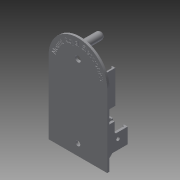
# Autodesk Inventor part: Robot Chassis(V2)7.stl
Saved by Autodesk Inventor 2015 SP1 (Build 190203100, 203)
## iProperties
Created: 2014-11-28
Part Number: Robot Chassis(V2)7.stl
Material: Generic
Document SubType Name: Modeling
Designer: shmyrk
Density: 1 g/cm^3
Appearance: Default
Author: shmyrk
Autodesk Inventor part; units mm, degrees
ref_plane "YZ Plane" through (0, 0, 0) normal (1, 0, 0) x (0, 1, 0)
ref_plane "XZ Plane" through (0, 0, 0) normal (0, 1, 0) x (-1, 0, 0)
ref_plane "XY Plane" through (0, 0, 0) normal (0, 0, 1) x (1, 0, 0)
sketch "Sketch1" plane through (0, 0, 0) normal (0, 1, 0) x (-1, 0, 0)
  line L0 (0, 0) -> (80, 0)
  line L1 (80, 0) -> (80, 100)
  line L2 (0, 100) -> (0, 0)
  arc A0 (80, 100) -> (0, 100) centre (40, 100) ccw
  dimension "d1" = 100
  dimension "d178" = 40
  dimension "d179" = 100
  dimension "d180" = 80
  constraints: 6 end point, 2 point on circle, 1 centre point, 1 horizontal, 1 parallel, 1 perpendicular
  measures "d1" distance of L1.end L0.end
  measures "d178" radius of A0
  measures "d179" distance from line of L0 A0.centre
  measures "d180" distance of L0.start L0.end
extrude "Extrusion1" add sketch "Sketch1" along normal blind 3
sketch "Sketch2" plane through (0, 3, 0) normal (0, 1, 0) x (1, 0, 0)
  line L0 (-80, -20) -> (-77, -20)
  line L1 (-77, -20) -> (-77, -56)
  line L2 (-77, -56) -> (-80, -56)
  line L3 (-80, -56) -> (-80, -20)
  line L4 (-3, -20) -> (0, -20)
  line L5 (0, -20) -> (0, -56)
  line L6 (0, -56) -> (-3, -56)
  line L7 (-3, -56) -> (-3, -20)
  line L8 (-77, -20) -> (-58, -20)
  line L9 (-3, -20) -> (-22, -20)
  line L10 (-58, -20) -> (-55, -20)
  line L11 (-55, -20) -> (-55, -56)
  line L12 (-55, -56) -> (-58, -56)
  line L13 (-58, -56) -> (-58, -20)
  line L14 (-25, -20) -> (-22, -20)
  line L15 (-22, -20) -> (-22, -56)
  line L16 (-22, -56) -> (-25, -56)
  line L17 (-25, -56) -> (-25, -20)
  line L18 (-80, -20) -> (-80, -20)
  line L19 (-80, 0) -> (-80, -100) projected
  line L20 (-80, -20) -> (-80, 0)
  line L21 (-80, 0) -> (-80, -100) projected
  line L22 (0, 0) -> (0, -100)
  arc A0 (-80, -100) -> (0, -100) centre (-40, -100) ccw projected
  line L23 (0, -20) -> (0, -20)
  dimension "d5" = 3
  dimension "d7" = 3
  dimension "d9" = 19
  dimension "d10" = 19
  dimension "d11" = 3
  dimension "d13" = 3
  dimension "d117" = 0
  dimension "d118" = 20
  dimension "d120" = 0
  dimension "d126" = 36
  constraints: 44 end point, 8 parallel, 6 collinear, 6 perpendicular, 5 horizontal, 2 point on line, 1 coincident, 1 tangent, 1 vertical
  measures "d5" distance of L1.end L2.end
  measures "d7" distance of L5.end L6.end
  measures "d9" distance of L8.end L0.end
  measures "d10" distance of L9.end L4.start
  measures "d11" distance of L11.end L12.end
  measures "d13" distance of L16.start L16.end
  measures "d117" distance of L0.start L18.end
  measures "d118" distance of L18.end L19.start
  measures "d120" distance of L23.start L4.end
  measures "d126" distance of L16.end L17.end
extrude "Extrusion2" add sketch "Sketch2" along normal blind 7
sketch "Sketch3" plane through (0, 10, 0) normal (0, 1, 0) x (1, 0, 0)
  line L0 (-80, -20) -> (-77, -20)
  line L1 (-77, -20) -> (-77, -41)
  line L2 (-77, -41) -> (-80, -41)
  line L3 (-80, -41) -> (-80, -20)
  line L4 (-3, -20) -> (0, -20)
  line L5 (0, -20) -> (0, -41)
  line L6 (0, -41) -> (-3, -41)
  line L7 (-3, -41) -> (-3, -20)
  line L8 (-58, -20) -> (-55, -20)
  line L9 (-55, -20) -> (-55, -41)
  line L10 (-55, -41) -> (-58, -41)
  line L11 (-58, -41) -> (-58, -20)
  line L12 (-25, -20) -> (-22, -20)
  line L13 (-22, -20) -> (-22, -41)
  line L14 (-22, -41) -> (-25, -41)
  line L15 (-25, -41) -> (-25, -20)
  point P0 (0, 0)
  dimension "d17" = 21
  dimension "d18" = 21
  dimension "d21" = 21
  dimension "d22" = 21
  constraints: 32 end point, 8 coincident, 8 parallel, 4 horizontal, 4 perpendicular
  measures "d17" distance of L0.end L1.end
  measures "d18" distance of L4.end L5.end
  measures "d21" distance of L8.end L9.end
  measures "d22" distance of L12.end L13.end
extrude "Extrusion3" add sketch "Sketch3" along normal blind 18
sketch "Sketch5" plane through (-77, 3, 56) normal (1, 0, 0) x (0, 0, -1)
  line L0 (15.017837, 25) -> (36, 25)
  line L1 (15, 25) -> (36, 25)
  line L2 (36, 25) -> (36, 23)
  line L3 (36, 23) -> (15, 23)
  line L4 (15, 23) -> (15, 25)
  point P0 (56, -3)
  point P1 (36, 25)
  dimension "d116" = 21
  dimension "d127" = 2
  constraints: 10 end point, 2 parallel, 1 coincident, 1 horizontal, 1 perpendicular, 1 point on line
  measures "d116" distance of L2.end L3.end
  measures "d127" distance of L3.end L1.start
sketch "Sketch6" plane through (-22, 3, 56) normal (1, 0, 0) x (0, 0, -1)
  line L0 (36, 0) -> (36, 25) projected
  line L1 (15, 25) -> (36, 25)
  line L2 (36, 25) -> (36, 23)
  line L3 (36, 23) -> (15, 23)
  line L4 (15, 23) -> (15, 25)
  point P0 (56, -3)
  constraints: 8 end point, 2 parallel, 1 horizontal, 1 perpendicular, 1 point on line
sketch "Sketch7" plane through (-3, 3, 20) normal (-1, 0, 0) x (0, 0, 1)
  line L0 (21, 7) -> (21, 25) projected
  line L1 (0, 25) -> (21, 25)
  line L2 (21, 25) -> (21, 23)
  line L3 (21, 23) -> (0, 23)
  line L4 (0, 23) -> (0, 25)
  point P0 (-20, -3)
  constraints: 8 end point, 2 parallel, 1 horizontal, 1 perpendicular, 1 point on line
sketch "Sketch8" plane through (-58, 3, 20) normal (-1, 0, 0) x (0, 0, 1)
  line L0 (21, 7) -> (21, 25) projected
  line L1 (0, 25) -> (21, 25)
  line L2 (21, 25) -> (21, 23)
  line L3 (21, 23) -> (0, 23)
  line L4 (0, 23) -> (0, 25)
  point P0 (-20, -3)
  constraints: 8 end point, 2 parallel, 1 horizontal, 1 perpendicular, 1 point on line
extrude "Extrusion4" add sketch "Sketch8" along normal blind 2
extrude "Extrusion5" add sketch "Sketch7" along normal blind 2
extrude "Extrusion6" add sketch "Sketch5" along normal blind 2
extrude "Extrusion7" add sketch "Sketch6" along normal blind 2
sketch "Sketch10" plane through (-80, 0, 0) normal (-1, 0, 0) x (0, 0, 1)
  circle A0 centre (33, 15) radius 2.5
  line L0 (33, 15) -> (33, 28)
  line L1 (33, 15) -> (41, 15)
  line L2 (20, 28) -> (41, 28) projected
  line L3 (33, 28) -> (41, 28)
  line L4 (41, 15) -> (41, 28)
  line L5 (41, 10) -> (41, 28) projected
  dimension "d36" = 5
  dimension "d128" = 8
  dimension "d130" = 13
  constraints: 8 end point, 1 centre point, 1 collinear, 1 horizontal, 1 point on line, 1 vertical
  measures "d36" diameter of A0
  measures "d128" distance of L0.start L1.end
  measures "d130" distance of L0.start L0.end
extrude "Extrusion8" cut sketch "Sketch10" against normal blind 5 contours L1 L0 A0 | A0 L0 L1
sketch "Sketch29" plane through (0, 0, 100) normal (1, 0, 0) x (0, 0, -1)
  line L0 (59, 15) -> (59, 28)
  line L1 (59, 15) -> (67, 15)
  line L2 (80, 28) -> (67, 28)
  line L3 (59, 28) -> (67, 28)
  line L4 (67, 15) -> (67, 28)
  line L5 (67, 23.946604) -> (67, 28)
  circle A0 centre (67, 15) radius 2.5
  point P0 (100, 0)
  dimension "d132" = 8
  dimension "d133" = 13
  dimension "d134" = 5
  constraints: 12 end point, 4 coincident, 1 centre point, 1 collinear, 1 horizontal, 1 perpendicular, 1 point on line, 1 vertical
  measures "d132" distance of L0.start L1.end
  measures "d133" distance of L0.start L0.end
  measures "d134" diameter of A0
extrude "Extrusion26" cut sketch "Sketch29" against normal blind 6 contours A0 L4 L1 | L1 L4 A0
sketch "Sketch11" plane through (0, 3, 0) normal (0, 1, 0) x (1, 0, 0)
  arc A0 (-40, -123) -> (-40, -133) centre (-40, -128) ccw
  line L0 (-80, -100) -> (0, -100)
  line L1 (-40, -100) -> (-40, -139.817705)
  arc A1 (-40, -133) -> (-40, -123) centre (-40, -128) ccw
  line L2 (-40, -128) -> (-80, -128)
  line L3 (-80, -128) -> (-80, -100)
  arc A2 (-80, -100) -> (0, -100) centre (-40, -100) ccw
  dimension "d41" = 10
  dimension "d138" = 28
  constraints: 8 end point, 4 point on circle, 3 point on line, 2 centre point, 2 horizontal, 1 coincident, 1 midpoint, 1 perpendicular, 1 tangent, 1 vertical
  measures "d41" diameter of A0
  measures "d138" distance of L2.end L0.start
extrude "Extrusion10" add sketch "Sketch11" along normal blind 25 contours L1 L2 A0 | A1 L1 | L2 L1 A0
sketch "Sketch12" plane through (-40, 28, 128) normal (0, 1, 0) x (1, 0, 0)
  circle A0 centre (0, 0) radius 5
  circle A1 centre (0, 0) radius 5
  line L0 (-0.004952, -4.999998) -> (0.052649, 4.999723)
  point P0 (40, 128)
  constraints: 4 point on circle, 2 end point, 1 centre point, 1 coincident, 1 concentric
revolve "Revolution1" add sketch "Sketch12" angle 180 about axis through (-40.004952, 28, 132.999998) along (0.0057602, 0, -0.9999834) picked at (-2.816726, -0.043754) contours L0 A0
sketch "Sketch13" plane through (0, 3, 0) normal (0, 1, 0) x (1, 0, 0)
  circle A0 centre (-40, -115) radius 4
  line L0 (-40, -115) -> (-40, -140)
  arc A1 (-80, -100) -> (0, -100) centre (-40, -100) ccw
  line L1 (-40, -115) -> (-2.919008, -115)
  line L2 (-40, -115) -> (-77.080992, -115)
  dimension "d45" = 8
  dimension "d177" = 25
  constraints: 6 end point, 3 point on circle, 1 centre point, 1 perpendicular, 1 point on line, 1 vertical
  measures "d45" diameter of A0
  measures "d177" distance of L0.start L0.end
extrude "Extrusion11" cut sketch "Sketch13" against normal blind 4 contours L1 L2 A0 | A0 L0 L1 | L2 L0 A0
sketch "Sketch18" plane through (0, 0, 0) normal (0, -1, 0) x (1, 0, 0)
  arc A0 (0, 100) -> (-80, 100) centre (-40, 100) ccw
  circle A1 centre (-40, 100) radius 30.265492
  line L0 (-68.738152, 109.835366) -> (-68.931541, 109.061765)
  line L1 (-68.931541, 109.061765) -> (-73.945796, 110.315251)
  line L2 (-73.945796, 110.315251) -> (-70.915049, 107.943792)
  line L3 (-70.915049, 107.943792) -> (-71.032969, 107.472084)
  line L4 (-71.032969, 107.472084) -> (-74.819581, 106.819895)
  line L5 (-74.819581, 106.819895) -> (-69.805325, 105.566408)
  line L6 (-69.805325, 105.566408) -> (-69.985742, 104.844695)
  line L7 (-69.985742, 104.844695) -> (-75.806619, 106.299824)
  line L8 (-75.806619, 106.299824) -> (-75.542479, 107.35645)
  line L9 (-75.542479, 107.35645) -> (-71.938652, 107.999202)
  line L10 (-71.938652, 107.999202) -> (-74.827886, 110.215)
  line L11 (-74.827886, 110.215) -> (-74.559029, 111.290494)
  line L12 (-74.559029, 111.290494) -> (-68.738152, 109.835366)
  spline S0 degree 2 poles (-68.817927, 115.195579) (-67.780675, 114.728018) (-67.099913, 113.221138) (-67.47556, 112.38779) knots 0 0 0 1 2 2 2
  spline S1 degree 2 poles (-67.47556, 112.38779) (-67.861198, 111.532279) (-69.468584, 111.078158) (-70.470375, 111.529734) knots 0 0 0 1 2 2 2
  spline S2 degree 2 poles (-70.470375, 111.529734) (-71.498762, 111.993299) (-72.182394, 113.517473) (-71.810743, 114.341955) knots 0 0 0 1 2 2 2
  spline S3 degree 2 poles (-71.810743, 114.341955) (-71.435096, 115.175303) (-69.850746, 115.661142) (-68.817927, 115.195579) knots 0 0 0 1 2 2 2
  spline S4 degree 2 poles (-69.139625, 114.481914) (-69.937511, 114.841576) (-70.974988, 114.610564) (-71.216761, 114.074207) knots 0 0 0 1 2 2 2
  spline S5 degree 2 poles (-71.216761, 114.074207) (-71.458534, 113.53785) (-70.946564, 112.603061) (-70.148677, 112.243399) knots 0 0 0 1 2 2 2
  spline S6 degree 2 poles (-70.148677, 112.243399) (-69.372954, 111.893727) (-68.311316, 112.119182) (-68.069543, 112.655539) knots 0 0 0 1 2 2 2
  spline S7 degree 2 poles (-68.069543, 112.655539) (-67.829768, 113.187463) (-68.350604, 114.126248) (-69.139625, 114.481914) knots 0 0 0 1 2 2 2
  line L13 (-64.479187, 117.883884) -> (-64.890533, 117.246601)
  line L14 (-64.890533, 117.246601) -> (-65.307218, 117.515557)
  spline S8 degree 2 poles (-65.307218, 117.515557) (-65.239706, 117.055306) (-65.314322, 116.356927) (-65.525269, 116.030115) knots 0 0 0 1 2 2 2
  spline S9 degree 2 poles (-65.525269, 116.030115) (-65.683479, 115.785006) (-66.129026, 115.453368) (-66.407524, 115.407431) knots 0 0 0 1 2 2 2
  spline S10 degree 2 poles (-66.407524, 115.407431) (-66.688658, 115.357409) (-67.339834, 115.523087) (-67.723838, 115.770949) knots 0 0 0 1 2 2 2
  line L15 (-67.723838, 115.770949) -> (-70.179014, 117.355685)
  line L16 (-70.179014, 117.355685) -> (-69.767669, 117.992969)
  line L17 (-69.767669, 117.992969) -> (-67.610708, 116.600722)
  spline S11 degree 2 poles (-67.610708, 116.600722) (-67.308407, 116.405596) (-66.883142, 116.19476) (-66.685977, 116.177452) knots 0 0 0 1 2 2 2
  spline S12 degree 2 poles (-66.685977, 116.177452) (-66.488812, 116.160144) (-66.182608, 116.338663) (-66.021761, 116.587858) knots 0 0 0 1 2 2 2
  spline S13 degree 2 poles (-66.021761, 116.587858) (-65.871462, 116.820711) (-65.796845, 117.51909) (-65.846458, 117.863619) knots 0 0 0 1 2 2 2
  line L18 (-65.846458, 117.863619) -> (-68.673383, 119.688307)
  line L19 (-68.673383, 119.688307) -> (-68.262038, 120.32559)
  line L20 (-68.262038, 120.32559) -> (-64.479187, 117.883884)
  line L21 (-61.473198, 121.402944) -> (-61.976117, 120.835134)
  line L22 (-61.976117, 120.835134) -> (-63.897935, 122.537323)
  spline S14 degree 2 poles (-63.897935, 122.537323) (-64.130883, 122.743648) (-64.569947, 123.054593) (-64.74809, 123.095464) knots 0 0 0 1 2 2 2
  spline S15 degree 2 poles (-64.74809, 123.095464) (-64.936736, 123.139142) (-65.279711, 123.001246) (-65.466694, 122.790137) knots 0 0 0 1 2 2 2
  spline S16 degree 2 poles (-65.466694, 122.790137) (-65.653677, 122.579028) (-65.824541, 121.931454) (-65.832758, 121.555513) knots 0 0 0 1 2 2 2
  line L23 (-65.832758, 121.555513) -> (-63.314012, 119.324614)
  line L24 (-63.314012, 119.324614) -> (-63.816931, 118.756805)
  line L25 (-63.816931, 118.756805) -> (-67.187392, 121.742082)
  line L26 (-67.187392, 121.742082) -> (-66.684472, 122.309892)
  line L27 (-66.684472, 122.309892) -> (-66.309572, 121.977836)
  spline S17 degree 2 poles (-66.309572, 121.977836) (-66.313211, 122.435725) (-66.11822, 123.139872) (-65.873208, 123.416498) knots 0 0 0 1 2 2 2
  spline S18 degree 2 poles (-65.873208, 123.416498) (-65.434765, 123.911511) (-64.283128, 123.89175) (-63.660721, 123.340473) knots 0 0 0 1 2 2 2
  line L28 (-63.660721, 123.340473) -> (-61.473198, 121.402944)
  spline S19 degree 2 poles (-59.603718, 122.949621) (-60.066128, 122.540367) (-61.054052, 122.607502) (-61.559979, 123.179143) knots 0 0 0 1 2 2 2
  line L29 (-61.559979, 123.179143) -> (-63.213106, 125.046986)
  line L30 (-63.213106, 125.046986) -> (-63.595414, 124.708627)
  line L31 (-63.595414, 124.708627) -> (-64.011112, 125.178319)
  line L32 (-64.011112, 125.178319) -> (-63.628805, 125.516678)
  line L33 (-63.628805, 125.516678) -> (-64.485982, 126.48519)
  line L34 (-64.485982, 126.48519) -> (-63.917983, 126.987895)
  line L35 (-63.917983, 126.987895) -> (-63.060806, 126.019383)
  line L36 (-63.060806, 126.019383) -> (-62.015833, 126.944232)
  line L37 (-62.015833, 126.944232) -> (-61.600134, 126.474541)
  line L38 (-61.600134, 126.474541) -> (-62.645107, 125.549692)
  line L39 (-62.645107, 125.549692) -> (-61.223998, 123.944001)
  spline S20 degree 2 poles (-61.223998, 123.944001) (-60.998425, 123.68913) (-60.73209, 123.424884) (-60.563851, 123.359512) knots 0 0 0 1 2 2 2
  spline S21 degree 2 poles (-60.563851, 123.359512) (-60.419425, 123.299037) (-60.096589, 123.396463) (-59.899974, 123.570476) knots 0 0 0 1 2 2 2
  spline S22 degree 2 poles (-59.899974, 123.570476) (-59.761615, 123.69293) (-59.577219, 124.005469) (-59.54152, 124.082516) knots 0 0 0 1 2 2 2
  line L40 (-59.54152, 124.082516) -> (-59.508751, 124.111518)
  line L41 (-59.508751, 124.111518) -> (-59.057605, 123.601775)
  spline S23 degree 2 poles (-59.057605, 123.601775) (-59.179141, 123.416294) (-59.461718, 123.075297) (-59.603718, 122.949621) knots 0 0 0 1 2 2 2
  line L42 (-52.410069, 127.73505) -> (-53.314226, 127.22999)
  line L43 (-53.314226, 127.22999) -> (-56.133969, 128.389463)
  line L44 (-56.133969, 128.389463) -> (-56.932004, 127.943682)
  line L45 (-56.932004, 127.943682) -> (-55.767758, 125.859453)
  line L46 (-55.767758, 125.859453) -> (-56.463917, 125.470581)
  line L47 (-56.463917, 125.470581) -> (-59.389943, 130.708746)
  line L48 (-59.389943, 130.708746) -> (-58.040075, 131.462779)
  spline S24 degree 2 poles (-58.040075, 131.462779) (-57.590119, 131.714123) (-56.928566, 131.955569) (-56.553061, 131.93141) knots 0 0 0 1 2 2 2
  spline S25 degree 2 poles (-56.553061, 131.93141) (-56.177555, 131.907252) (-55.548567, 131.529013) (-55.318563, 131.11726) knots 0 0 0 1 2 2 2
  spline S26 degree 2 poles (-55.318563, 131.11726) (-54.998455, 130.544204) (-55.150322, 129.440171) (-55.546885, 128.973599) knots 0 0 0 1 2 2 2
  line L49 (-55.546885, 128.973599) -> (-52.410069, 127.73505)
  spline S27 degree 2 poles (-56.01361, 130.656607) (-56.141653, 130.88583) (-56.499766, 131.148049) (-56.733582, 131.167814) knots 0 0 0 1 2 2 2
  spline S28 degree 2 poles (-56.733582, 131.167814) (-56.936689, 131.182454) (-57.376514, 131.042588) (-57.665165, 130.881348) knots 0 0 0 1 2 2 2
  line L50 (-57.665165, 130.881348) -> (-58.357078, 130.494847)
  line L51 (-58.357078, 130.494847) -> (-57.256854, 128.525229)
  line L52 (-57.256854, 128.525229) -> (-56.645594, 128.866678)
  spline S29 degree 2 poles (-56.645594, 128.866678) (-56.344208, 129.035031) (-55.923818, 129.409095) (-55.850743, 129.667121) knots 0 0 0 1 2 2 2
  spline S30 degree 2 poles (-55.850743, 129.667121) (-55.778548, 129.896808) (-55.861855, 130.384935) (-56.01361, 130.656607) knots 0 0 0 1 2 2 2
  spline S31 degree 2 poles (-49.298462, 131.223663) (-48.907053, 130.155344) (-49.507747, 128.614796) (-50.366054, 128.30033) knots 0 0 0 1 2 2 2
  spline S32 degree 2 poles (-50.366054, 128.30033) (-51.247188, 127.977501) (-52.696073, 128.808554) (-53.074101, 129.840349) knots 0 0 0 1 2 2 2
  spline S33 degree 2 poles (-53.074101, 129.840349) (-53.462165, 130.899536) (-52.85112, 132.454234) (-52.001944, 132.765354) knots 0 0 0 1 2 2 2
  spline S34 degree 2 poles (-52.001944, 132.765354) (-51.143637, 133.079819) (-49.688199, 132.287416) (-49.298462, 131.223663) knots 0 0 0 1 2 2 2
  spline S35 degree 2 poles (-50.033502, 130.95436) (-50.334586, 131.776143) (-51.225382, 132.355977) (-51.777804, 132.153582) knots 0 0 0 1 2 2 2
  spline S36 degree 2 poles (-51.777804, 132.153582) (-52.330225, 131.951186) (-52.640145, 130.931435) (-52.339061, 130.109652) knots 0 0 0 1 2 2 2
  spline S37 degree 2 poles (-52.339061, 130.109652) (-52.04634, 129.310696) (-51.142615, 128.709707) (-50.590194, 128.912103) knots 0 0 0 1 2 2 2
  spline S38 degree 2 poles (-50.590194, 128.912103) (-50.042338, 129.112825) (-49.735763, 130.141707) (-50.033502, 130.95436) knots 0 0 0 1 2 2 2
  line L53 (-45.247633, 134.429517) -> (-46.334411, 127.900103)
  line L54 (-46.334411, 127.900103) -> (-47.128638, 127.731174)
  line L55 (-47.128638, 127.731174) -> (-46.729626, 129.734849)
  line L56 (-46.729626, 129.734849) -> (-49.218768, 133.584872)
  line L57 (-49.218768, 133.584872) -> (-48.419785, 133.754813)
  line L58 (-48.419785, 133.754813) -> (-46.522631, 130.748222)
  line L59 (-46.522631, 130.748222) -> (-46.018081, 134.265646)
  line L60 (-46.018081, 134.265646) -> (-45.247633, 134.429517)
  spline S39 degree 2 poles (-41.270971, 130.728663) (-41.358339, 130.654266) (-41.651664, 130.389881) (-41.792043, 130.306874) knots 0 0 0 1 2 2 2
  spline S40 degree 2 poles (-41.792043, 130.306874) (-41.983382, 130.186156) (-42.348987, 130.048284) (-42.688502, 130.024359) knots 0 0 0 1 2 2 2
  spline S41 degree 2 poles (-42.688502, 130.024359) (-42.964964, 130.004877) (-43.479232, 130.178232) (-43.68172, 130.35406) knots 0 0 0 1 2 2 2
  spline S42 degree 2 poles (-43.68172, 130.35406) (-43.874166, 130.525722) (-44.130705, 131.053565) (-44.151896, 131.354278) knots 0 0 0 1 2 2 2
  spline S43 degree 2 poles (-44.151896, 131.354278) (-44.184708, 131.819898) (-43.838324, 132.507211) (-43.424835, 132.726447) knots 0 0 0 1 2 2 2
  spline S44 degree 2 poles (-43.424835, 132.726447) (-43.058823, 132.927714) (-42.039807, 133.131128) (-41.445624, 133.20712) knots 0 0 0 1 2 2 2
  line L61 (-41.445624, 133.20712) -> (-41.455877, 133.352626)
  spline S45 degree 2 poles (-41.455877, 133.352626) (-41.474334, 133.614537) (-41.65729, 133.928222) (-41.809291, 134.010122) knots 0 0 0 1 2 2 2
  spline S46 degree 2 poles (-41.809291, 134.010122) (-41.961291, 134.092023) (-42.38251, 134.120832) (-42.60562, 134.105109) knots 0 0 0 1 2 2 2
  spline S47 degree 2 poles (-42.60562, 134.105109) (-42.867531, 134.086653) (-43.564725, 133.881545) (-43.908194, 133.706238) knots 0 0 0 1 2 2 2
  line L62 (-43.908194, 133.706238) -> (-43.951846, 133.703162)
  line L63 (-43.951846, 133.703162) -> (-44.006191, 134.474346)
  spline S48 degree 2 poles (-44.006191, 134.474346) (-43.801733, 134.547245) (-43.031103, 134.747779) (-42.647936, 134.77478) knots 0 0 0 1 2 2 2
  spline S49 degree 2 poles (-42.647936, 134.77478) (-42.182316, 134.807592) (-41.536685, 134.706859) (-41.271145, 134.535474) knots 0 0 0 1 2 2 2
  spline S50 degree 2 poles (-41.271145, 134.535474) (-41.010796, 134.368597) (-40.726929, 133.798812) (-40.697194, 133.376843) knots 0 0 0 1 2 2 2
  line L64 (-40.697194, 133.376843) -> (-40.480843, 130.306661)
  line L65 (-40.480843, 130.306661) -> (-41.237475, 130.253342)
  line L66 (-41.237475, 130.253342) -> (-41.270971, 130.728663)
  line L67 (-41.315403, 131.35919) -> (-41.403242, 132.605694)
  spline S51 degree 2 poles (-41.403242, 132.605694) (-41.673145, 132.562302) (-42.48702, 132.422087) (-42.738612, 132.326369) knots 0 0 0 1 2 2 2
  spline S52 degree 2 poles (-42.738612, 132.326369) (-43.032831, 132.213024) (-43.398697, 131.802173) (-43.374772, 131.462658) knots 0 0 0 1 2 2 2
  spline S53 degree 2 poles (-43.374772, 131.462658) (-43.347429, 131.074641) (-42.883225, 130.712535) (-42.466108, 130.741929) knots 0 0 0 1 2 2 2
  spline S54 degree 2 poles (-42.466108, 130.741929) (-42.112042, 130.766879) (-41.55155, 131.113457) (-41.315403, 131.35919) knots 0 0 0 1 2 2 2
  line L68 (-38.644949, 130.237521) -> (-39.403063, 130.261981)
  line L69 (-39.403063, 130.261981) -> (-39.200953, 136.526145)
  line L70 (-39.200953, 136.526145) -> (-38.442838, 136.501685)
  line L71 (-38.442838, 136.501685) -> (-38.644949, 130.237521)
  line L72 (-34.916382, 129.884268) -> (-33.578757, 135.733265)
  line L73 (-33.578757, 135.733265) -> (-29.919579, 134.896436)
  line L74 (-29.919579, 134.896436) -> (-30.077839, 134.204415)
  line L75 (-30.077839, 134.204415) -> (-32.959679, 134.863472)
  line L76 (-32.959679, 134.863472) -> (-33.326062, 133.261397)
  line L77 (-33.326062, 133.261397) -> (-30.638558, 132.646783)
  line L78 (-30.638558, 132.646783) -> (-30.796818, 131.954762)
  line L79 (-30.796818, 131.954762) -> (-33.484323, 132.569376)
  line L80 (-33.484323, 132.569376) -> (-33.980783, 130.398517)
  line L81 (-33.980783, 130.398517) -> (-31.098944, 129.73946)
  line L82 (-31.098944, 129.73946) -> (-31.257204, 129.047439)
  line L83 (-31.257204, 129.047439) -> (-34.916382, 129.884268)
  line L84 (-29.768186, 128.486028) -> (-30.485199, 128.733472)
  line L85 (-30.485199, 128.733472) -> (-28.44062, 134.658021)
  line L86 (-28.44062, 134.658021) -> (-27.723607, 134.410578)
  line L87 (-27.723607, 134.410578) -> (-29.768186, 128.486028)
  spline S55 degree 2 poles (-26.984861, 127.212991) (-27.96372, 127.667938) (-28.529304, 129.265878) (-28.057962, 130.280011) knots 0 0 0 1 2 2 2
  spline S56 degree 2 poles (-28.057962, 130.280011) (-27.594818, 131.276506) (-26.000606, 131.972504) (-25.158435, 131.581086) knots 0 0 0 1 2 2 2
  spline S57 degree 2 poles (-25.158435, 131.581086) (-24.779238, 131.404846) (-24.29527, 130.911824) (-24.187829, 130.577716) knots 0 0 0 1 2 2 2
  spline S58 degree 2 poles (-24.187829, 130.577716) (-24.075979, 130.241559) (-24.155832, 129.458327) (-24.383305, 128.968898) knots 0 0 0 1 2 2 2
  line L88 (-24.383305, 128.968898) -> (-24.557497, 128.59411)
  line L89 (-24.557497, 128.59411) -> (-27.38384, 129.907718)
  spline S59 degree 2 poles (-27.38384, 129.907718) (-27.713779, 129.197825) (-27.349909, 128.111851) (-26.714974, 127.816751) knots 0 0 0 1 2 2 2
  spline S60 degree 2 poles (-26.714974, 127.816751) (-26.490101, 127.712236) (-26.006449, 127.610767) (-25.79319, 127.608162) knots 0 0 0 1 2 2 2
  spline S61 degree 2 poles (-25.79319, 127.608162) (-25.567015, 127.610276) (-25.239551, 127.645741) (-25.122986, 127.677352) knots 0 0 0 1 2 2 2
  line L90 (-25.122986, 127.677352) -> (-25.083303, 127.658909)
  line L91 (-25.083303, 127.658909) -> (-25.431685, 126.909332)
  spline S62 degree 2 poles (-25.431685, 126.909332) (-25.573278, 126.916162) (-26.000416, 126.943108) (-26.159957, 126.969003) knots 0 0 0 1 2 2 2
  spline S63 degree 2 poles (-26.159957, 126.969003) (-26.385015, 127.003901) (-26.737942, 127.09823) (-26.984861, 127.212991) knots 0 0 0 1 2 2 2
  spline S64 degree 2 poles (-24.983838, 129.430308) (-24.86355, 129.712191) (-24.789655, 130.171126) (-24.836358, 130.359046) knots 0 0 0 1 2 2 2
  spline S65 degree 2 poles (-24.836358, 130.359046) (-24.883683, 130.568702) (-25.182646, 130.906037) (-25.46043, 131.035143) knots 0 0 0 1 2 2 2
  spline S66 degree 2 poles (-25.46043, 131.035143) (-25.733805, 131.1622) (-26.193236, 131.177347) (-26.425745, 131.092389) knots 0 0 0 1 2 2 2
  spline S67 degree 2 poles (-26.425745, 131.092389) (-26.655894, 131.000971) (-26.997016, 130.682321) (-27.139972, 130.432421) knots 0 0 0 1 2 2 2
  line L92 (-27.139972, 130.432421) -> (-24.983838, 129.430308)
  spline S68 degree 2 poles (-23.369269, 125.168193) (-23.762375, 125.419881) (-24.258774, 126.078334) (-24.334876, 126.473464) knots 0 0 0 1 2 2 2
  spline S69 degree 2 poles (-24.334876, 126.473464) (-24.4136, 126.8645) (-24.194419, 127.774933) (-23.874566, 128.274505) knots 0 0 0 1 2 2 2
  spline S70 degree 2 poles (-23.874566, 128.274505) (-23.554714, 128.774077) (-22.821878, 129.332547) (-22.439357, 129.434043) knots 0 0 0 1 2 2 2
  spline S71 degree 2 poles (-22.439357, 129.434043) (-22.054214, 129.539633) (-21.21634, 129.378454) (-20.831424, 129.132011) knots 0 0 0 1 2 2 2
  spline S72 degree 2 poles (-20.831424, 129.132011) (-20.520215, 128.932758) (-20.051481, 128.384393) (-19.899672, 128.125541) knots 0 0 0 1 2 2 2
  line L93 (-19.899672, 128.125541) -> (-20.358477, 127.408942)
  line L94 (-20.358477, 127.408942) -> (-20.395331, 127.432537)
  spline S73 degree 2 poles (-20.395331, 127.432537) (-20.428239, 127.534435) (-20.546789, 127.81818) (-20.648485, 127.992987) knots 0 0 0 1 2 2 2
  spline S74 degree 2 poles (-20.648485, 127.992987) (-20.741667, 128.145022) (-21.036471, 128.478106) (-21.200265, 128.582976) knots 0 0 0 1 2 2 2
  spline S75 degree 2 poles (-21.200265, 128.582976) (-21.695742, 128.900207) (-22.777464, 128.536245) (-23.215295, 127.852404) knots 0 0 0 1 2 2 2
  spline S76 degree 2 poles (-23.215295, 127.852404) (-23.642639, 127.184943) (-23.540948, 126.063298) (-23.024997, 125.732959) knots 0 0 0 1 2 2 2
  spline S77 degree 2 poles (-23.024997, 125.732959) (-22.713788, 125.533706) (-21.983529, 125.429882) (-21.638036, 125.491577) knots 0 0 0 1 2 2 2
  line L95 (-21.638036, 125.491577) -> (-21.601183, 125.467981)
  line L96 (-21.601183, 125.467981) -> (-22.059987, 124.751382)
  spline S78 degree 2 poles (-22.059987, 124.751382) (-22.183008, 124.766639) (-22.550922, 124.82322) (-22.68393, 124.867965) knots 0 0 0 1 2 2 2
  spline S79 degree 2 poles (-22.68393, 124.867965) (-22.879185, 124.923697) (-23.168621, 125.039728) (-23.369269, 125.168193) knots 0 0 0 1 2 2 2
  spline S80 degree 2 poles (-20.66084, 123.172996) (-21.141809, 123.560269) (-21.24121, 124.545469) (-20.762456, 125.140053) knots 0 0 0 1 2 2 2
  line L97 (-20.762456, 125.140053) -> (-19.198118, 127.082865)
  line L98 (-19.198118, 127.082865) -> (-19.59577, 127.403051)
  line L99 (-19.59577, 127.403051) -> (-19.202398, 127.891594)
  line L100 (-19.202398, 127.891594) -> (-18.804747, 127.571408)
  line L101 (-18.804747, 127.571408) -> (-17.993609, 128.578792)
  line L102 (-17.993609, 128.578792) -> (-17.402812, 128.103087)
  line L103 (-17.402812, 128.103087) -> (-18.21395, 127.095703)
  line L104 (-18.21395, 127.095703) -> (-17.127036, 126.220527)
  line L105 (-17.127036, 126.220527) -> (-17.520408, 125.731984)
  line L106 (-17.520408, 125.731984) -> (-18.607322, 126.60716)
  line L107 (-18.607322, 126.60716) -> (-19.952103, 124.937023)
  spline S81 degree 2 poles (-19.952103, 124.937023) (-20.165561, 124.671922) (-20.381428, 124.365064) (-20.417676, 124.188248) knots 0 0 0 1 2 2 2
  spline S82 degree 2 poles (-20.417676, 124.188248) (-20.453088, 124.035729) (-20.30293, 123.73379) (-20.098423, 123.569123) knots 0 0 0 1 2 2 2
  spline S83 degree 2 poles (-20.098423, 123.569123) (-19.954511, 123.453246) (-19.615487, 123.323844) (-19.533547, 123.301564) knots 0 0 0 1 2 2 2
  line L108 (-19.533547, 123.301564) -> (-19.499463, 123.274119)
  line L109 (-19.499463, 123.274119) -> (-19.926377, 122.743917)
  spline S84 degree 2 poles (-19.926377, 122.743917) (-20.129605, 122.832645) (-20.513141, 123.05407) (-20.66084, 123.172996) knots 0 0 0 1 2 2 2
  line L110 (-15.260883, 123.304092) -> (-15.288738, 123.331243)
  spline S85 degree 2 poles (-15.288738, 123.331243) (-15.334441, 123.409742) (-15.463443, 123.549067) (-15.557451, 123.640702) knots 0 0 0 1 2 2 2
  spline S86 degree 2 poles (-15.557451, 123.640702) (-15.776804, 123.854517) (-16.395211, 124.08386) (-16.773461, 124.085901) knots 0 0 0 1 2 2 2
  line L111 (-16.773461, 124.085901) -> (-19.003243, 121.798362)
  line L112 (-19.003243, 121.798362) -> (-19.546403, 122.327808)
  line L113 (-19.546403, 122.327808) -> (-16.403666, 125.551949)
  line L114 (-16.403666, 125.551949) -> (-15.860506, 125.022503)
  line L115 (-15.860506, 125.022503) -> (-16.328862, 124.542016)
  spline S87 degree 2 poles (-16.328862, 124.542016) (-15.774974, 124.518152) (-15.122365, 124.303) (-14.913458, 124.099367) knots 0 0 0 1 2 2 2
  spline S88 degree 2 poles (-14.913458, 124.099367) (-14.829895, 124.017913) (-14.753119, 123.929497) (-14.711074, 123.868143) knots 0 0 0 1 2 2 2
  line L116 (-14.711074, 123.868143) -> (-15.260883, 123.304092)
  spline S89 degree 2 poles (-13.361668, 118.75574) (-14.249774, 118.044562) (-15.901406, 118.123508) (-16.472779, 118.837029) knots 0 0 0 1 2 2 2
  spline S90 degree 2 poles (-16.472779, 118.837029) (-17.059349, 119.569527) (-16.732847, 121.207608) (-15.875104, 121.894472) knots 0 0 0 1 2 2 2
  spline S91 degree 2 poles (-15.875104, 121.894472) (-14.994589, 122.599572) (-13.326249, 122.515318) (-12.760953, 121.809388) knots 0 0 0 1 2 2 2
  spline S92 degree 2 poles (-12.760953, 121.809388) (-12.18958, 121.095867) (-12.477358, 119.463879) (-13.361668, 118.75574) knots 0 0 0 1 2 2 2
  spline S93 degree 2 poles (-13.850983, 119.366787) (-13.167824, 119.913847) (-12.901781, 120.942898) (-13.269527, 121.402132) knots 0 0 0 1 2 2 2
  spline S94 degree 2 poles (-13.269527, 121.402132) (-13.637272, 121.861366) (-14.702631, 121.830485) (-15.385789, 121.283425) knots 0 0 0 1 2 2 2
  spline S95 degree 2 poles (-15.385789, 121.283425) (-16.049971, 120.751562) (-16.331952, 119.703519) (-15.964206, 119.244285) knots 0 0 0 1 2 2 2
  spline S96 degree 2 poles (-15.964206, 119.244285) (-15.5995, 118.788846) (-14.52655, 118.825806) (-13.850983, 119.366787) knots 0 0 0 1 2 2 2
  line L117 (-12.923353, 113.639628) -> (-13.303874, 114.295783)
  line L118 (-13.303874, 114.295783) -> (-11.083041, 115.5837)
  spline S97 degree 2 poles (-11.083041, 115.5837) (-10.813849, 115.739811) (-10.380446, 116.0586) (-10.285551, 116.214805) knots 0 0 0 1 2 2 2
  spline S98 degree 2 poles (-10.285551, 116.214805) (-10.184682, 116.380095) (-10.207542, 116.749045) (-10.349017, 116.993) knots 0 0 0 1 2 2 2
  spline S99 degree 2 poles (-10.349017, 116.993) (-10.490493, 117.236955) (-11.051299, 117.603076) (-11.40552, 117.729275) knots 0 0 0 1 2 2 2
  line L119 (-11.40552, 117.729275) -> (-14.316157, 116.041324)
  line L120 (-14.316157, 116.041324) -> (-14.696678, 116.697479)
  line L121 (-14.696678, 116.697479) -> (-10.801808, 118.956212)
  line L122 (-10.801808, 118.956212) -> (-10.421287, 118.300057)
  line L123 (-10.421287, 118.300057) -> (-10.854518, 118.048815)
  spline S100 degree 2 poles (-10.854518, 118.048815) (-10.418785, 117.908059) (-9.811884, 117.501222) (-9.626502, 117.181556) knots 0 0 0 1 2 2 2
  spline S101 degree 2 poles (-9.626502, 117.181556) (-9.294766, 116.609523) (-9.676226, 115.522718) (-10.395473, 115.105609) knots 0 0 0 1 2 2 2
  line L124 (-10.395473, 115.105609) -> (-12.923353, 113.639628)
  line L125 (-12.192644, 111.95386) -> (-12.500914, 112.6469)
  line L126 (-12.500914, 112.6469) -> (-8.387096, 114.47676)
  line L127 (-8.387096, 114.47676) -> (-8.078825, 113.78372)
  line L128 (-8.078825, 113.78372) -> (-12.192644, 111.95386)
  line L129 (-7.372933, 114.03917) -> (-7.722701, 114.825504)
  line L130 (-7.722701, 114.825504) -> (-7.003005, 115.145631)
  line L131 (-7.003005, 115.145631) -> (-6.653237, 114.359296)
  line L132 (-6.653237, 114.359296) -> (-7.372933, 114.03917)
  spline S102 degree 2 poles (-11.272627, 109.206366) (-11.421477, 109.648772) (-11.396115, 110.472986) (-11.207991, 110.828695) knots 0 0 0 1 2 2 2
  spline S103 degree 2 poles (-11.207991, 110.828695) (-11.024476, 111.182854) (-10.283432, 111.755377) (-9.721209, 111.944541) knots 0 0 0 1 2 2 2
  spline S104 degree 2 poles (-9.721209, 111.944541) (-9.158986, 112.133704) (-8.237909, 112.110152) (-7.876127, 111.949722) knots 0 0 0 1 2 2 2
  spline S105 degree 2 poles (-7.876127, 111.949722) (-7.509737, 111.790843) (-6.957457, 111.140459) (-6.811708, 110.707271) knots 0 0 0 1 2 2 2
  spline S106 degree 2 poles (-6.811708, 110.707271) (-6.693868, 110.357034) (-6.671855, 109.63597) (-6.715611, 109.339094) knots 0 0 0 1 2 2 2
  line L133 (-6.715611, 109.339094) -> (-7.522079, 109.067753)
  line L134 (-7.522079, 109.067753) -> (-7.536034, 109.109229)
  spline S107 degree 2 poles (-7.536034, 109.109229) (-7.497875, 109.209278) (-7.4126, 109.504733) (-7.38241, 109.704704) knots 0 0 0 1 2 2 2
  spline S108 degree 2 poles (-7.38241, 109.704704) (-7.359843, 109.881589) (-7.381079, 110.32589) (-7.4431, 110.510225) knots 0 0 0 1 2 2 2
  spline S109 degree 2 poles (-7.4431, 110.510225) (-7.630713, 111.06784) (-8.701975, 111.461528) (-9.471575, 111.202591) knots 0 0 0 1 2 2 2
  spline S110 degree 2 poles (-9.471575, 111.202591) (-10.222742, 110.949856) (-10.845903, 110.011719) (-10.650538, 109.431063) knots 0 0 0 1 2 2 2
  spline S111 degree 2 poles (-10.650538, 109.431063) (-10.532698, 109.080825) (-10.028398, 108.542551) (-9.720409, 108.374282) knots 0 0 0 1 2 2 2
  line L135 (-9.720409, 108.374282) -> (-9.706454, 108.332806)
  line L136 (-9.706454, 108.332806) -> (-10.512922, 108.061465)
  spline S112 degree 2 poles (-10.512922, 108.061465) (-10.599276, 108.150402) (-10.850673, 108.424923) (-10.926346, 108.543104) knots 0 0 0 1 2 2 2
  spline S113 degree 2 poles (-10.926346, 108.543104) (-11.043668, 108.708833) (-11.196651, 108.980556) (-11.272627, 109.206366) knots 0 0 0 1 2 2 2
  spline S114 degree 2 poles (-10.463775, 106.095373) (-10.55406, 106.538457) (-10.472143, 107.354055) (-10.390194, 107.633747) knots 0 0 0 1 2 2 2
  line L137 (-10.390194, 107.633747) -> (-9.556436, 107.803638)
  line L138 (-9.556436, 107.803638) -> (-9.548669, 107.765523)
  spline S115 degree 2 poles (-9.548669, 107.765523) (-9.605483, 107.654704) (-9.734104, 107.360539) (-9.790469, 107.125757) knots 0 0 0 1 2 2 2
  spline S116 degree 2 poles (-9.790469, 107.125757) (-9.843129, 106.921503) (-9.883333, 106.436944) (-9.833822, 106.193963) knots 0 0 0 1 2 2 2
  spline S117 degree 2 poles (-9.833822, 106.193963) (-9.797902, 106.017683) (-9.63439, 105.629218) (-9.548273, 105.547523) knots 0 0 0 1 2 2 2
  spline S118 degree 2 poles (-9.548273, 105.547523) (-9.429598, 105.427802) (-9.19949, 105.345674) (-8.98986, 105.38839) knots 0 0 0 1 2 2 2
  spline S119 degree 2 poles (-8.98986, 105.38839) (-8.727821, 105.441784) (-8.514503, 105.78298) (-8.498732, 106.168279) knots 0 0 0 1 2 2 2
  spline S120 degree 2 poles (-8.498732, 106.168279) (-8.494506, 106.318005) (-8.492417, 106.794797) (-8.479812, 107.000814) knots 0 0 0 1 2 2 2
  spline S121 degree 2 poles (-8.479812, 107.000814) (-8.435023, 107.535928) (-7.918386, 108.117567) (-7.484832, 108.205911) knots 0 0 0 1 2 2 2
  spline S122 degree 2 poles (-7.484832, 108.205911) (-6.884525, 108.328232) (-5.953043, 107.58019) (-5.801597, 106.836954) knots 0 0 0 1 2 2 2
  spline S123 degree 2 poles (-5.801597, 106.836954) (-5.726845, 106.4701) (-5.756444, 105.689973) (-5.843156, 105.40931) knots 0 0 0 1 2 2 2
  line L139 (-5.843156, 105.40931) -> (-6.6388, 105.247185)
  line L140 (-6.6388, 105.247185) -> (-6.646567, 105.2853)
  spline S124 degree 2 poles (-6.646567, 105.2853) (-6.476127, 105.617759) (-6.355826, 106.366746) (-6.428637, 106.724071) knots 0 0 0 1 2 2 2
  spline S125 degree 2 poles (-6.428637, 106.724071) (-6.503389, 107.090925) (-6.915976, 107.532842) (-7.225658, 107.469739) knots 0 0 0 1 2 2 2
  spline S126 degree 2 poles (-7.225658, 107.469739) (-7.506754, 107.412462) (-7.71716, 107.056973) (-7.734962, 106.705995) knots 0 0 0 1 2 2 2
  spline S127 degree 2 poles (-7.734962, 106.705995) (-7.744833, 106.53527) (-7.747102, 106.108063) (-7.753882, 105.87346) knots 0 0 0 1 2 2 2
  spline S128 degree 2 poles (-7.753882, 105.87346) (-7.778732, 105.362257) (-8.244724, 104.751241) (-8.73545, 104.651248) knots 0 0 0 1 2 2 2
  spline S129 degree 2 poles (-8.73545, 104.651248) (-9.02131, 104.592999) (-9.571958, 104.714017) (-9.802424, 104.895315) knots 0 0 0 1 2 2 2
  spline S130 degree 2 poles (-9.802424, 104.895315) (-10.045331, 105.088965) (-10.371548, 105.642762) (-10.463775, 106.095373) knots 0 0 0 1 2 2 2
  constraints: 1 centre point, 1 coincident, 1 other
emboss "Emboss1" sketch "Sketch18" operation cut depth 1 direction (0, 1, 0) contours L68 L69 L70 L71 | L83 L72 L73 L74 L75 L76 L77 L78 L79 L80 L81 L82 | L112 L113 L114 L115 S87 S88 L116 L110 S85 S86 L111 | S130 S114 A1 | A1 S114 L137 L138 S115 S116 S117 S118 S119 S120 S121 S122 S123 L139 L140 S124 S125 S126 S127 S128 S129 S130 | S1 S2 S3 S0 A1 | A1 S0 S1 | S113 S102 A1 | A1 S102 S103 S104 S105 S106 L133 L134 S107 S108 S109 S110 S111 L135 L136 S112 S113 | S9 S10 L15 L16 L17 S11 S12 S13 L18 L19 L20 L13 L14 S8 A1 | A1 S8 S9 | S89 S90 A1 | A1 S90 S91 S92 S89 | S19 L29 L30 L31 L32 L33 L34 L35 L36 L37 L38 L39 S20 S21 S22 L40 L41 S23 A1 | A1 S23 S19 | S32 S33 S34 S31 A1 | A1 S31 S32 | S84 S80 A1 | A1 S80 L97 L98 L99 L100 L101 L102 L103 L104 L105 L106 L107 S81 S82 S83 L108 L109 S84 | L55 L56 L57 L58 L59 L60 L53 A1 | A1 L53 L54 L55 | S79 S68 A1 | A1 S68 S69 S70 S71 S72 L93 L94 S73 S74 S75 S76 S77 L95 L96 S78 S79 | S41 S42 S43 S44 L61 S45 S46 S47 L62 L63 S48 S49 S50 L64 L65 L66 S39 S40 A1 | A1 S40 S41 | S63 S55 A1 | A1 S55 S56 S57 S58 L88 L89 S59 S60 S61 L90 L91 S62 S63 | L0 L1 L2 L3 L4 L5 L6 L7 L8 L9 L10 L11 L12 | L21 L22 S14 S15 S16 L23 L24 L25 L26 L27 S17 S18 L28 | L42 L43 L44 L45 L46 L47 L48 S24 S25 S26 L49 | L84 L85 L86 L87 | L117 L118 S97 S98 S99 L119 L120 L121 L122 L123 S100 S101 L124 | L125 L126 L127 L128 | L129 L130 L131 L132
sketch "Sketch19" plane through (0, 3, 0) normal (0, 1, 0) x (1, 0, 0)
  arc A0 (-80, -100) -> (0, -100) centre (-40, -100) ccw projected
  line L0 (-22, -56) -> (-25, -56) projected
  line L1 (-55, -56) -> (-55, -63) construction
  line L2 (-40, -100) -> (-40, -63) construction
  line L3 (-40, -63) -> (-39, -63) construction
  line L4 (-41, -63) -> (-40, -63) construction
  line L5 (-39, -63) -> (-39, -108)
  line L6 (-41, -63) -> (-41, -108)
  line L7 (-39, -63) -> (-41, -63)
  line L8 (-39, -108) -> (-41, -108)
  line L9 (-39, -63) -> (-13, -63) construction
  line L10 (-41, -63) -> (-67, -63) construction
  line L11 (-68, -100) -> (-68, -63) construction
  line L12 (-68, -63) -> (-67, -63) construction
  line L13 (-69, -63) -> (-68, -63) construction
  line L14 (-67, -63) -> (-67, -108)
  line L15 (-69, -63) -> (-69, -108)
  line L16 (-67, -63) -> (-69, -63)
  line L17 (-67, -108) -> (-69, -108)
  line L18 (-12, -100) -> (-12, -63) construction
  line L19 (-12, -63) -> (-11, -63) construction
  line L20 (-13, -63) -> (-12, -63) construction
  line L21 (-11, -63) -> (-11, -108)
  line L22 (-13, -63) -> (-13, -108)
  line L23 (-11, -63) -> (-13, -63)
  line L24 (-11, -108) -> (-13, -108)
  dimension "d73" = 7
  dimension "d78" = 1
  dimension "d79" = 1
  dimension "d80" = 45
  dimension "d81" = 45
  dimension "d82" = 26
  dimension "d83" = 26
  dimension "d84" = 1
  dimension "d85" = 1
  dimension "d86" = 45
  dimension "d87" = 45
  dimension "d88" = 1
  dimension "d89" = 1
  dimension "d90" = 45
  dimension "d91" = 45
  constraints: 48 end point, 10 perpendicular, 5 parallel, 1 collinear
  measures "d73" distance of L1.start L1.end
  measures "d78" distance of L2.end L3.end
  measures "d79" distance of L4.start L4.end
  measures "d80" distance of L3.end L5.end
  measures "d81" distance of L6.start L6.end
  measures "d82" distance of L3.end L9.end
  measures "d83" distance of L6.start L10.end
  measures "d84" distance of L12.start L12.end
  measures "d85" distance of L13.start L13.end
  measures "d86" distance of L12.end L14.end
  measures "d87" distance of L16.end L15.end
  measures "d88" distance of L18.end L21.start
  measures "d89" distance of L20.start L20.end
  measures "d90" distance of L21.start L21.end
  measures "d91" distance of L22.start L22.end
extrude "Extrusion16" add sketch "Sketch19" along normal blind 19
sketch "Sketch20" plane through (0, 3, 0) normal (0, 1, 0) x (1, 0, 0)
  line L0 (-22, -56) -> (-25, -56) projected
  line L1 (-69, -63) -> (-69, -62)
  line L2 (-69, -62) -> (-11, -62)
  line L3 (-11, -62) -> (-11, -63)
  line L4 (-69, -63) -> (-11, -63)
  line L5 (-69, -109) -> (-69, -108)
  line L6 (-69, -108) -> (-11, -108)
  line L7 (-11, -108) -> (-11, -109)
  line L8 (-69, -109) -> (-11, -109)
  dimension "d94" = 1
  dimension "d95" = 1
  constraints: 16 end point, 4 parallel, 3 perpendicular
  measures "d94" distance of L1.start L1.end
  measures "d95" distance of L8.start L6.start
extrude "Extrusion17" add sketch "Sketch20" along normal blind 3
sketch "Sketch21" plane through (-67, 22, 108) normal (1, 0, 0) x (0, 0, -1)
  line L0 (45, -16) -> (45, 0) projected
  line L1 (0, 0) -> (45, 0) projected
  line L2 (0, -16) -> (0, 0) projected
  line L3 (0, 0) -> (0, -2)
  line L4 (0, -2) -> (45, -2)
  line L5 (45, 0) -> (0, 0)
  point P0 (108, -22)
  dimension "d98" = 2
  constraints: 6 end point, 2 point on line, 1 collinear, 1 perpendicular
  measures "d98" distance of L1.start L3.end
sketch "Sketch24" plane through (-13, 22, 63) normal (-1, 0, 0) x (0, 0, 1)
  line L0 (45, -16) -> (45, 0) projected
  line L1 (0, 0) -> (45, 0) projected
  line L2 (0, -16) -> (0, 0) projected
  line L3 (0, 0) -> (0, -2)
  line L4 (0, -2) -> (45, -2)
  line L5 (45, 0) -> (0, 0)
  point P0 (-63, -22)
  dimension "d99" = 2
  constraints: 6 end point, 2 point on line, 1 collinear, 1 perpendicular
  measures "d99" distance of L1.start L3.end
sketch "Sketch25" plane through (-41, 22, 63) normal (-1, 0, 0) x (0, 0, 1)
  line L0 (45, -16) -> (45, 0) projected
  line L1 (0, 0) -> (45, 0)
  line L2 (45, 0) -> (45, -2)
  line L3 (45, -2) -> (0, -2)
  line L4 (0, -2) -> (0, 0)
  point P0 (-63, -22)
  constraints: 8 end point, 2 parallel, 1 horizontal, 1 perpendicular, 1 point on line
sketch "Sketch26" plane through (-39, 22, 108) normal (1, 0, 0) x (0, 0, -1)
  line L0 (45, -16) -> (45, 0) projected
  line L1 (0, 0) -> (45, 0)
  line L2 (45, 0) -> (45, -2)
  line L3 (45, -2) -> (0, -2)
  line L4 (0, -2) -> (0, 0)
  point P0 (108, -22)
  constraints: 8 end point, 2 parallel, 1 horizontal, 1 perpendicular, 1 point on line
extrude "Extrusion22" add sketch "Sketch26" along normal blind 2
extrude "Extrusion23" add sketch "Sketch21" along normal blind 2
extrude "Extrusion24" add sketch "Sketch24" along normal blind 2
extrude "Extrusion25" add sketch "Sketch25" along normal blind 2
chamfer "Chamfer1" distance 2.75 distance2 6.25 1 edges at (-40, 3, 133) measured on face at (-40, 3, 133.5)
sketch "Sketch30" plane through (0, 0, 0) normal (0, -1, 0) x (1, 0, 0)
  circle A0 centre (-40, 15) radius 3.25
  line L0 (0, 0) -> (-80, 0) projected
  line L1 (-40, 0) -> (-40, 15)
  line L2 (-40, 15) -> (0, 15)
  line L3 (0, 100) -> (0, 0) projected
  line L4 (-40, 15) -> (-80, 15)
  line L5 (-80, 0) -> (-80, 100) projected
  dimension "d142" = 6.5
  dimension "d143" = 15
  dimension "d144" = 40
  constraints: 6 end point, 2 horizontal, 2 point on line, 1 centre point, 1 midpoint, 1 perpendicular
  measures "d142" diameter of A0
  measures "d143" distance of L1.start L1.end
  measures "d144" distance of L1.end L2.end
extrude "Extrusion27" cut sketch "Sketch30" against normal blind 7 contours L2 L4 A0 | A0 L1 L2 | L4 L1 A0
chamfer "Chamfer2" distance 2.75 distance2 3.75 1 edges at (-25, 3, 38) measured on face at (-25.5, 3, 38)
chamfer "Chamfer3" distance 2.75 distance2 3.75 1 edges at (-55, 3, 38) measured on face at (-54.5, 3, 38)
chamfer "Chamfer4" distance 2 distance2 2 1 edges at (-78.5, 10, 41) measured on face at (-78.5, 10, 41.5)
chamfer "Chamfer5" distance 2 distance2 2 1 edges at (-56.5, 10, 41) measured on face at (-56.5, 10, 41.5)
chamfer "Chamfer6" distance 2 distance2 2 1 edges at (-23.5, 10, 41) measured on face at (-23.5, 10, 41.5)
chamfer "Chamfer7" distance 2 distance2 2 1 edges at (-1.5, 10, 41) measured on face at (-1.5, 10, 41.5)
chamfer "Chamfer8" distance 4 distance2 4 1 edges at (-1.5, 3, 20) measured on face at (-1.5, 3, 19.5)
chamfer "Chamfer9" distance 4 distance2 4 2 edges at (-26.375, 3, 20) (-23.5, 3, 20) measured on face at (-23.5, 3, 19.5) measured on face at (-26.375, 3, 19.5)
chamfer "Chamfer10" distance 4 distance2 4 2 edges at (-53.625, 3, 20) (-56.5, 3, 20) measured on face at (-56.5, 3, 19.5) measured on face at (-53.625, 3, 19.5)
chamfer "Chamfer11" distance 4 distance2 4 1 edges at (-78.5, 3, 20) measured on face at (-78.5, 3, 19.5)
body "Solid1"
